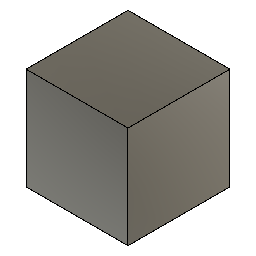
cube (Autodesk Fusion 360 design; units mm, degrees)
Autodesk Fusion 360 part; units mm, degrees
box "Grundkörper Quader1" add length 20 width 20 height 20 placed x (0, -1, 0) y (1, 0, 0) z (0, 0, 1) at (-10, 10, 0)
